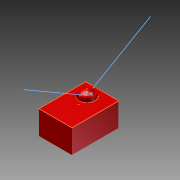
# Autodesk Inventor part: Camera
Saved by Autodesk Inventor 2011 (Build 150239000, 239)
## iProperties
Created: 2011-01-28
Part Number: Camera
Document SubType Name: Modeling
Designer: Physics Student
Density: 1.4 g/cm^3
Material: PVC-Piping
Mass: 109.493 g
Surface Area: 115.717 cm^2
Volume: 78.2096 cm^3
Author: Physics Student
Autodesk Inventor part; units mm, degrees
ref_plane "YZ Plane" through (0, 0, 0) normal (1, 0, 0) x (0, 1, 0)
ref_plane "XZ Plane" through (0, 0, 0) normal (0, 1, 0) x (-1, 0, 0)
sketch "Sketch1" plane through (0, 0, 0) normal (0, 0, 1) x (1, 0, 0)
  line L0 (-21.1, 29.81) -> (21.1, 29.81)
  line L1 (21.1, 29.81) -> (21.1, -29.81)
  line L2 (21.1, -29.81) -> (-21.1, -29.81)
  line L3 (-21.1, -29.81) -> (-21.1, 29.81)
  line L4 (0, 0) -> (0, 68.2086)
  line L5 (0, 0) -> (53.7664, 0)
  dimension "d0" = 59.62
  dimension "d1" = 42.2
  constraints: 12 end point, 3 parallel, 2 perpendicular, 1 horizontal, 2 other
  measures "d0" distance between parallel lines of L2 L0
  measures "d1" distance between parallel lines of L1 L3
extrude "Extrusion1" add sketch "Sketch1" along normal blind 30.3
ref_plane "Work Plane1" through (-3.92, -29.81, 0) normal (-1, 0, 0) x (0, 0, 1)
sketch "Sketch3" plane through (-3.92, -29.81, 0) normal (-1, 0, 0) x (0, 0, 1)
  line L0 (0, 59.62) -> (30.3, 59.62) projected
  line L1 (30.3, 59.62) -> (30.3, 0) projected
  line L2 (30.3, 44.35) -> (38.03, 44.35)
  line L3 (39.0073, 54.42) -> (18.3537, 54.42)
  arc A0 (30.3, 34.28) -> (30.3, 54.42) centre (27.6058, 44.35) ccw
  point P0 (0, 29.81)
  dimension "d8" = 7.73
  dimension "d9" = 15.27
  dimension "d10" = 5.2
  dimension "d11" = 20.14
  constraints: 4 end point, 4 point on line, 3 point on circle, 1 centre point, 1 parallel, 1 perpendicular
  measures "d8" distance of L2.start L2.end
  measures "d9" distance between parallel lines of L0 L2
  measures "d10" distance between parallel lines of L0 L3
  measures "d11" distance of A0.end A0.start
revolve "Revolution1" add sketch "Sketch3" angle 360 about axis through (-3.92, 14.54, 30.3) along (0, 0, 1) picked at (31.0054, 37.9107) contours L2 A0 L1
sketch "Sketch6" plane through (0, 0, 30.3) normal (0, 0, 1) x (1, 0, 0)
  circle A0 centre (-3.92, 14.54) radius 10.07 projected
  circle A1 centre (-3.92, 14.54) radius 10.07
  point P0 (0, 0)
  constraints: 1 centre point, 1 coincident, 1 concentric
extrude "Extrusion4" add sketch "Sketch6" along normal blind 5.43
sketch "Sketch7" plane through (21.1, -29.81, 0) normal (1, 0, 0) x (0, 0, -1)
  line L0 (-35.73, 34.28) -> (-35.73, 54.42) projected
  line L1 (-35.73, 54.42) -> (-46.1148, 54.42)
  line L2 (-46.1148, 54.42) -> (-46.1148, 34.28)
  line L3 (-46.1148, 34.28) -> (-35.73, 34.28)
  line L4 (-35.73, 34.28) -> (-35.73, 54.42)
  point P0 (0, 29.81)
  constraints: 8 end point, 2 parallel, 1 horizontal, 1 perpendicular
extrude "Extrusion5" cut sketch "Sketch7" against normal blind 400
sketch "Sketch8" plane through (-3.92, -29.81, 0) normal (-1, 0, 0) x (0, 0, 1)
  line L0 (35.73, 54.42) -> (35.73, 34.28) projected
  line L1 (35.73, 44.35) -> (38.6, 44.35)
  line L2 (31.2686, 37.15) -> (43.7794, 37.15)
  line L3 (30.3, 34.28) -> (35.73, 34.28) projected
  line L4 (31.2686, 51.55) -> (47.0475, 51.55)
  line L5 (30.3, 54.42) -> (35.73, 54.42) projected
  arc A0 (35.73, 37.15) -> (35.73, 51.55) centre (28.1336, 44.35) ccw
  point P0 (0, 29.81)
  dimension "d27" = 2.87
  dimension "d28" = 2.87
  dimension "d29" = 2.87
  constraints: 6 end point, 4 point on line, 3 point on circle, 2 parallel, 1 centre point, 1 midpoint, 1 perpendicular
  measures "d27" distance between parallel lines of L3 L2
  measures "d28" distance between parallel lines of L5 L4
  measures "d29" distance of L1.start L1.end
revolve "Revolution2" add sketch "Sketch8" angle 360 about axis through (-3.92, 14.54, 35.73) along (0, 0, 1) picked at (36.137, 48.6296) contours A0 L1 L0
sketch "Sketch9" plane through (-3.92, -29.81, 0) normal (-1, 0, 0) x (0, 0, 1)
  line L0 (35.73, 54.42) -> (35.73, 34.28) projected
  line L1 (30.3, 54.42) -> (30.3, 34.28) projected
  line L2 (35.73, 51.55) -> (35.73, 37.15) projected
  line L3 (31.5731, 44.35) -> (78.5809, 125.77)
  line L4 (31.5731, 44.35) -> (78.5809, -37.07)
  line L5 (30.3, 44.35) -> (31.5731, 44.35) construction
  point P0 (0, 29.81)
  point P1 (38.6, 44.35)
  dimension "d31" = 120
  constraints: 6 end point, 2 point on line, 1 equal length, 1 midpoint, 1 perpendicular
  measures "d31" angle of L3 L4
sketch "Sketch10" plane through (0, 0, 30.3) normal (0, 0, 1) x (1, 0, 0)
  circle A0 centre (-3.92, 14.54) radius 10.07 projected
  line L0 (21.1, 29.81) -> (21.1, -29.81) projected
  line L1 (-21.1, 29.81) -> (21.1, 29.81) projected
  line L2 (-21.1, -29.81) -> (-21.1, 29.81) projected
  line L3 (21.1, -29.81) -> (-21.1, -29.81) projected
  point P0 (0, 0)
body "Solid1"
